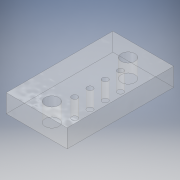
# Autodesk Inventor part: phone_holder_side_cap
Saved by Autodesk Inventor 2019 (Build 230136000, 136)
## iProperties
Created: 2019-02-17
Part Number: phone_holder_side_cap
Material: Acrylic, Clear
Document SubType Name: Modeling
Designer: suchanek
Density: 1.19 g/cm^3
Appearance: Transparent - Clear
Author: suchanek
Autodesk Inventor part; units mm, degrees
ref_plane "YZ Plane" through (0, 0, 0) normal (1, 0, 0) x (0, 1, 0)
ref_plane "XZ Plane" through (0, 0, 0) normal (0, 1, 0) x (-1, 0, 0)
ref_plane "XY Plane" through (0, 0, 0) normal (0, 0, 1) x (1, 0, 0)
sketch "Sketch2" plane through (0, 0, 0) normal (0, 1, 0) x (-1, 0, 0)
  line L0 (0, 0) -> (-20, 0)
  line L1 (-20, 0) -> (-20, 35)
  line L2 (-20, 35) -> (0, 35)
  line L3 (0, 35) -> (0, 0)
  circle A0 centre (-10, 5) radius 2.25
  circle A1 centre (-10, 30) radius 2.25
  circle A2 centre (-12.5, 10) radius 0.95
  circle A3 centre (-12.5, 15) radius 0.95
  circle A4 centre (-12.5, 20) radius 0.95
  circle A5 centre (-12.5, 25) radius 0.95
  dimension "d76" = 20
  dimension "d77" = 35
  dimension "d78" = 5
  dimension "d79" = 25
  dimension "d80" = 10
  dimension "d81" = 4.5
  dimension "d82" = 1.9
  dimension "d85" = 5
  dimension "d90" = 5
  dimension "d91" = 7.5
  constraints: 8 end point, 6 centre point, 2 parallel, 1 equal radius, 1 horizontal, 1 perpendicular, 1 vertical, 1 vertical alignment, 6 other
  measures "d76" distance of L1.end L2.end
  measures "d77" distance of L0.end L1.end
  measures "d78" distance from line of L0 A0.centre
  measures "d79" distance of A1.centre A0.centre
  measures "d80" distance from line of L3 A0.centre
  measures "d81" diameter of A1
  measures "d82" diameter of A2
  measures "d85" distance of A2.centre A3.centre
  measures "d90" vertical distance of A2.centre A0.centre
  measures "d91" distance from line of L1 A2.centre
extrude "Extrusion2" add sketch "Sketch2" along normal blind 6
body "Solid2"
